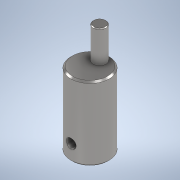
# Autodesk Inventor part: crankshaft valve crank
Saved by Autodesk Inventor 2020 (Build 240168000, 168)
## iProperties
Created: 2020-08-04
Part Number: crankshaft valve crank
Material: Stainless Steel
Document SubType Name: Modeling
Designer: benny
Density: 8 g/cm^3
Appearance: Semi-Polished
Author: benny
Autodesk Inventor part; units mm, degrees
ref_plane "YZ Plane" through (0, 0, 0) normal (1, 0, 0) x (0, 1, 0)
ref_plane "XZ Plane" through (0, 0, 0) normal (0, 1, 0) x (-1, 0, 0)
ref_plane "XY Plane" through (0, 0, 0) normal (0, 0, 1) x (1, 0, 0)
sketch "Sketch1" plane through (0, 0, 0) normal (0, 1, 0) x (-1, 0, 0)
  circle A0 centre (0, 0) radius 6
  dimension "d0" = 12
  constraints: 1 centre point, 1 coincident
  measures "d0" diameter of A0
extrude "Extrusion1" add sketch "Sketch1" along normal blind 22
sketch "Sketch2" plane through (0, 22, 0) normal (0, 1, 0) x (1, 0, 0)
  circle A0 centre (0, 0) radius 6
  dimension "d3" = 12
  constraints: 1 centre point, 1 coincident
  measures "d3" diameter of A0
extrude "Extrusion2" add sketch "Sketch2" along normal blind 0.5 draft -45
sketch "Sketch3" plane through (0, 0, 0) normal (0, -1, 0) x (1, 0, 0)
  circle A0 centre (0, 0) radius 6
  dimension "d6" = 12
  constraints: 1 centre point, 1 coincident
  measures "d6" diameter of A0
extrude "Extrusion3" add sketch "Sketch3" along normal blind 0.5 draft -45
sketch "Sketch6" plane through (0, 0, 0) normal (0, 0, 1) x (1, 0, 0)
  circle A0 centre (0, 4.5) radius 1.5
  point P0 (0, 0)
  dimension "d9" = 3
  constraints: 1 centre point
  measures "d9" diameter of A0
extrude "Extrusion4" cut sketch "Sketch6" along normal mid plane 12
sketch "Sketch7" plane through (0, 22.5, 0) normal (0, 1, 0) x (1, 0, 0)
  circle A0 centre (0, 3) radius 2
  point P0 (0, 0)
  dimension "d12" = 4
  constraints: 1 centre point
  measures "d12" diameter of A0
extrude "Extrusion5" add sketch "Sketch7" along normal blind 9.75
sketch "Sketch9" plane through (0, 32.25, -3) normal (0, 1, 0) x (1, 0, 0)
  circle A0 centre (0, 0) radius 2
  point P0 (0, -3)
  dimension "d15" = 4
  constraints: 1 centre point
  measures "d15" diameter of A0
extrude "Extrusion6" add sketch "Sketch9" along normal blind 0.25 draft -45
body "Solid1"
